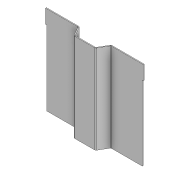
# Autodesk Inventor part: voetensteun v2
Saved by Autodesk Inventor 2020.3 (Build 243373000, 373)
## iProperties
Created: 2020-10-02
Part Number: voetensteun v2
Material: Generic
Document SubType Name: Sheet Metal
Designer: Svend
Density: 1 g/cm^3
Sheet Metal Rule: Default_mm
Appearance: Default
Author: Svend
Autodesk Inventor part; units mm, degrees
ref_plane "YZ Plane" through (0, 0, 0) normal (1, 0, 0) x (0, 1, 0)
ref_plane "XZ Plane" through (0, 0, 0) normal (0, 1, 0) x (-1, 0, 0)
ref_plane "XY Plane" through (0, 0, 0) normal (0, 0, 1) x (1, 0, 0)
sketch "Sketch1" plane through (0, 0, 0) normal (0, 0, 1) x (1, 0, 0)
  line L0 (-50, 205.75) -> (50, 205.75)
  line L1 (50, 205.75) -> (50, -205.75)
  line L2 (50, -205.75) -> (-50, -205.75)
  line L3 (-50, -205.75) -> (-50, 205.75)
  line L4 (-50, 205.75) -> (50, -205.75) construction
  line L5 (50, 205.75) -> (-50, -205.75) construction
  point P0 (0, 0)
  dimension "d0" = 411.5
  dimension "d1" = 100
  measures "d0" distance of L0.end L1.end
  measures "d1" distance of L0.start L0.end
extrude "Plate1" add sketch "Sketch1" along normal blind 4
sketch "Sketch2" plane through (-46.5359, 205.75, 2) normal (-0.8660254, 0, 0.5) x (0, -1, 0)
  line L0 (411.5, 0) -> (0, 0)
  line L1 (0, 0) -> (0, -55)
  line L2 (0, -55) -> (411.5, -55)
  line L3 (411.5, -55) -> (411.5, 0)
  constraints: 6 end point, 1 horizontal, 1 perpendicular, 1 vertical
edge flange "Flange1" height 55 angle 60 thickness 4 bend radius 4 thickness toward (-0.8660254, 0, 0.5) relief straight relief width 4 relief depth 2 edges at (-50, 0, 0) wall of the first edge with corners at (-46.5359, -205.75, 2) (-46.5359, 205.75, 2) (-74.0359, 205.75, -45.6314) (-74.0359, -205.75, -45.6314)
bend "Bend1"
corner "Corner1"
sketch "Sketch3" plane through (-74.0359, -205.75, -41.6314) normal (0, 0, -1) x (-1, 0, 0)
  line L0 (0, 411.5) -> (0, 0)
  line L1 (0, 0) -> (153, 0)
  line L2 (153, 0) -> (153, 411.5)
  line L3 (153, 411.5) -> (0, 411.5)
  constraints: 6 end point, 1 horizontal, 1 perpendicular, 1 vertical
edge flange "Flange2" height 153 angle 60 thickness 4 bend radius 4 thickness toward (0, 0, -1) relief straight relief width 4 relief depth 2 edges at (-77.5, 0, -43.6314) wall of the first edge with corners at (-74.0359, 205.75, -41.6314) (-74.0359, -205.75, -41.6314) (-227.0359, -205.75, -41.6314) (-227.0359, 205.75, -41.6314)
bend "Bend2"
corner "Corner2"
sketch "Sketch4" plane through (46.5359, -205.75, 2) normal (0.8660254, 0, 0.5) x (0, 1, 0)
  line L0 (411.5, 0) -> (0, 0)
  line L1 (0, 0) -> (0, -55)
  line L2 (0, -55) -> (411.5, -55)
  line L3 (411.5, -55) -> (411.5, 0)
  constraints: 6 end point, 1 horizontal, 1 perpendicular, 1 vertical
edge flange "Flange3" height 55 angle 60 thickness 4 bend radius 4 thickness toward (0.8660254, 0, 0.5) relief straight relief width 4 relief depth 2 edges at (50, 0, 0) wall of the first edge with corners at (46.5359, 205.75, 2) (46.5359, -205.75, 2) (74.0359, -205.75, -45.6314) (74.0359, 205.75, -45.6314)
bend "Bend3"
corner "Corner3"
sketch "Sketch5" plane through (74.0359, 205.75, -41.6314) normal (0, 0, -1) x (-1, 0, 0)
  line L0 (0, -411.5) -> (0, 0)
  line L1 (0, 0) -> (-153, 0)
  line L2 (-153, 0) -> (-153, -411.5)
  line L3 (-153, -411.5) -> (0, -411.5)
  constraints: 6 end point, 1 horizontal, 1 perpendicular, 1 vertical
edge flange "Flange4" height 153 angle 60 thickness 4 bend radius 4 thickness toward (0, 0, -1) relief straight relief width 4 relief depth 2 edges at (77.5, 0, -43.6314) wall of the first edge with corners at (74.0359, -205.75, -41.6314) (74.0359, 205.75, -41.6314) (227.0359, 205.75, -41.6314) (227.0359, -205.75, -41.6314)
bend "Bend4"
corner "Corner4"
sketch "Sketch6" plane through (-227.0359, -205.75, -45.6314) normal (0, 0, -1) x (-1, 0, 0)
  line L0 (-148.3812, 411.5) -> (-148.3812, 0) projected
  line L1 (0, 0) -> (-148.3812, 0) projected
  line L2 (0, 411.5) -> (0, 0) projected
  line L3 (-148.3812, 411.5) -> (0, 411.5) projected
  line L4 (-305.6906, 0) -> (-305.6906, 411.5) projected
  line L5 (-454.0718, 411.5) -> (-305.6906, 411.5) projected
  line L6 (-454.0718, 0) -> (-454.0718, 411.5) projected
  line L7 (-305.6906, 0) -> (-454.0718, 0) projected
  line L8 (-454.0718, 0) -> (-449.0718, 0)
  line L9 (-449.0718, 0) -> (-449.0718, 346.5)
  line L10 (-449.0718, 346.5) -> (-454.0718, 346.5)
  line L11 (-454.0718, 346.5) -> (-454.0718, 0)
  line L12 (-148.3812, 0) -> (0, 0) projected
  line L13 (0, 0) -> (-5, 0)
  line L14 (-5, 0) -> (-5, 346.5)
  line L15 (-5, 346.5) -> (0, 346.5)
  line L16 (0, 346.5) -> (0, 0)
  point P0 (-227.0359, 205.75)
  dimension "d43" = 5
  dimension "d46" = 65
  constraints: 16 end point, 4 parallel, 2 horizontal, 2 perpendicular, 1 collinear, 1 point on line
  measures "d43" distance of L9.end L10.end
  measures "d46" distance between parallel lines of L5 L10
extrude "Cut1" cut sketch "Sketch6" against normal blind 4 contours L14 L15 L2 L1 | L7 L6 L10 L9
equation "\"d44\" = Thickness"
equation "\"d2\" = Thickness"
equation "\"d3\" = BendReliefWidth"
equation "\"d4\" = BendReliefDepth"
equation "\"d5\" = MinimumRemnant"
equation "\"d6\" = TransitionRadius"
equation "\"d9\" = BendRadius"
equation "\"d10\" = CornerReliefSize"
equation "\"d11\" = GapSize"
equation "\"d12\" = JacobiRadiusSize"
equation "\"d13\" = BendReliefWidth"
equation "\"d14\" = BendReliefDepth"
equation "\"d15\" = MinimumRemnant"
equation "\"d16\" = TransitionRadius"
equation "\"d19\" = BendRadius"
equation "\"d20\" = CornerReliefSize"
equation "\"d21\" = GapSize"
equation "\"d22\" = JacobiRadiusSize"
equation "\"d23\" = BendReliefWidth"
equation "\"d24\" = BendReliefDepth"
equation "\"d25\" = MinimumRemnant"
equation "\"d26\" = TransitionRadius"
equation "\"d29\" = BendRadius"
equation "\"d30\" = CornerReliefSize"
equation "\"d31\" = GapSize"
equation "\"d32\" = JacobiRadiusSize"
equation "\"d33\" = BendReliefWidth"
equation "\"d34\" = BendReliefDepth"
equation "\"d35\" = MinimumRemnant"
equation "\"d36\" = TransitionRadius"
equation "\"d39\" = BendRadius"
equation "\"d40\" = CornerReliefSize"
equation "\"d41\" = GapSize"
equation "\"d42\" = JacobiRadiusSize"
equation "\"BendRadius\" = Thickness"
equation "\"BendReliefWidth\" = Thickness"
equation "\"BendReliefDepth\" = 0.5 * Thickness"
equation "\"CornerReliefSize\" = 4 * Thickness"
equation "\"MinimumRemnant\" = 2 * Thickness"
equation "\"TransitionRadius\" = BendRadius"
equation "\"JacobiRadiusSize\" = BendRadius"
equation "\"GapSize\" = Thickness"
equation "\"Thickness\" = 4"
body "Solid1"
